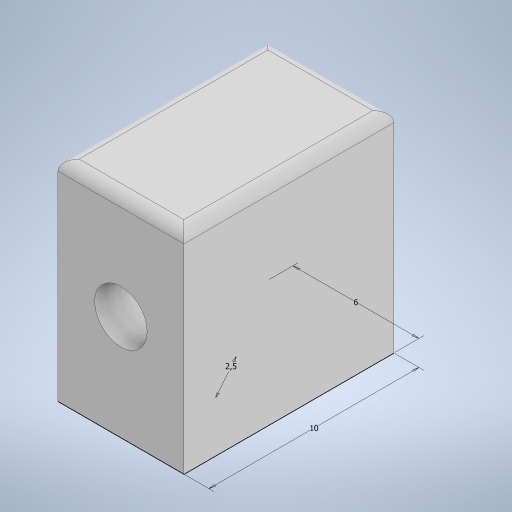
# Autodesk Inventor part: pusher
Saved by Autodesk Inventor 2023 (Build 270158000, 158)
## iProperties
Created: 2026-02-18
Part Number: pusher
Material: Типовые
Document SubType Name: Modeling
Designer: garin
Density: 1 g/cm^3
Appearance: По умолчанию
Author: garin
Autodesk Inventor part; units mm, degrees
ref_plane "YZ Plane" through (0, 0, 0) normal (1, 0, 0) x (0, 1, 0)
ref_plane "XZ Plane" through (0, 0, 0) normal (0, 1, 0) x (-1, 0, 0)
ref_plane "XY Plane" through (0, 0, 0) normal (0, 0, 1) x (1, 0, 0)
sketch "Эскиз2" plane through (0, 0, 0) normal (0, 1, 0) x (-1, 0, 0)
  line L0 (3, 5) -> (-3, 5)
  line L1 (-3, 5) -> (-3, -5)
  line L2 (-3, -5) -> (3, -5)
  line L3 (3, -5) -> (3, 5)
  line L4 (3, 0) -> (-3, 0) construction
  line L5 (0, 5) -> (0, -5) construction
  circle A0 centre (0, 0) radius 1.25
  dimension "d0" = 6
  dimension "d1" = 10
  dimension "d2" = 2.5
  constraints: 12 end point, 5 midpoint, 2 coincident, 2 parallel, 1 centre point, 1 horizontal, 1 perpendicular
  measures "d0" distance of L2.end L1.end
  measures "d1" distance of L1.end L0.end
  measures "d2" diameter of A0
extrude "Выдавливание1" add sketch "Эскиз2" along normal blind 10 contours L3 L2 L1 L0 | A0
sketch "Эскиз4" plane through (-3, 0, 5) normal (0, 0, 1) x (1, 0, 0)
  line L0 (3, 0) -> (3, 10) construction
  line L1 (6, 10) -> (0, 10) construction
  line L2 (0, 0) -> (0, 10) construction
  line L3 (0, 5) -> (6, 5) construction
  line L4 (6, 0) -> (6, 10) construction
  circle A0 centre (3, 5) radius 1.25
  dimension "d8" = 2.5
  constraints: 4 end point, 4 midpoint, 1 centre point
  measures "d8" diameter of A0
extrude "Выдавливание3" cut sketch "Эскиз4" against normal blind 10
fillet "Сопряжение1" radius 0.5 4 edges at (-3, 10, 0) (0, 10, 5) (3, 10, 0) (0, 10, -5)
